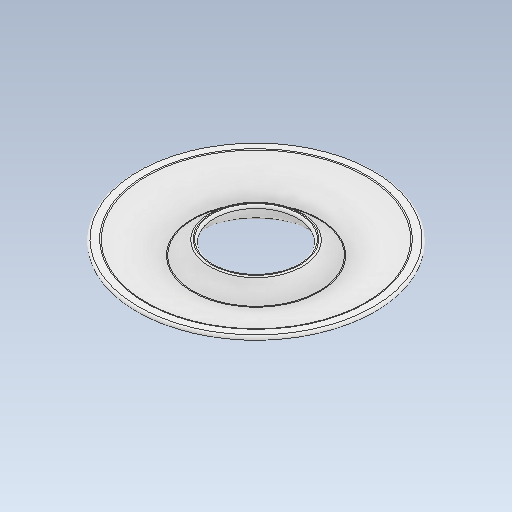
# Autodesk Inventor part: 8002_base_132uH_DCore_2layer_Tx_Filter_MPSv2_v1
Saved by Autodesk Inventor 2021 (Build 250183000, 183)
## iProperties
Created: 2021-02-24
Part Number: 8002_base_132uH_DCore_2layer_Tx_Filter_MPSv2_v1
Material: Acetal Resin, White
Document SubType Name: Modeling
Designer: Barksdale
Density: 1.425 g/cm^3
Appearance: Smooth - White
Author: Barksdale
Autodesk Inventor part; units mm, degrees
ref_plane "YZ Plane" through (0, 0, 0) normal (1, 0, 0) x (0, 1, 0)
ref_plane "XZ Plane" through (0, 0, 0) normal (0, 1, 0) x (-1, 0, 0)
ref_plane "XY Plane" through (0, 0, 0) normal (0, 0, 1) x (1, 0, 0)
sketch "Sketch1" plane through (0, 0, 0) normal (0, 0, 1) x (1, 0, 0)
  arc A0 (15.1396, -15.5997) -> (26.1298, -12.284) centre (15.0348, 4.6194) ccw
  arc A1 (11.0335, -12.4095) -> (14.937, -15.558) centre (18.7381, -6.8515) ccw
  arc A2 (9.9209, -12.8881) -> (14.937, -18.058) centre (18.7381, -9.3515) ccw
  arc A3 (15.1396, -18.0997) -> (28.3715, -13.0778) centre (15.0348, 2.1194) ccw
  line L0 (26.4042, -12.202) -> (28.0417, -12.202)
  line L1 (28.0417, -12.202) -> (26.2537, -12.202)
  line L2 (10.628, -12.202) -> (10.3849, -12.202)
  arc A4 (10.3849, -12.202) -> (9.9209, -12.8881) centre (10.3849, -12.702) ccw
  arc A5 (11.0335, -12.4095) -> (10.628, -12.202) centre (10.628, -12.702) ccw
  arc A6 (26.4042, -12.202) -> (26.1298, -12.284) centre (26.4042, -12.702) ccw
  arc A7 (28.3715, -13.0778) -> (28.0417, -12.202) centre (28.0417, -12.702) ccw
  arc A8 (14.937, -18.058) -> (15.1396, -18.0997) centre (15.137, -17.5997) ccw
  arc A9 (14.937, -15.558) -> (15.1396, -15.5997) centre (15.137, -15.0997) ccw
  line L3 (0, 0) -> (0, -18.0894)
  line L4 (15.137, -17.5997) -> (19.2939, -17.5997)
  line L5 (19.2939, -17.5997) -> (19.2939, -19.2305)
  line L6 (19.2939, -19.2305) -> (15.137, -19.2305)
  line L7 (15.137, -19.2305) -> (15.137, -17.5997)
  point P0 (9.6758, -12.202)
  point P1 (10.888, -12.202)
  point P2 (19.2939, -17.6463)
  point P3 (15.137, -18.0997)
  dimension "d1" = 0.5
  constraints: 23 point on circle, 16 end point, 12 tangent, 10 centre point, 5 equal radius, 3 point on line, 2 horizontal, 2 parallel, 1 perpendicular, 1 vertical
  measures "d1" radius of A4
revolve "Revolution2" add sketch "Sketch1" angle 360 about axis through (0, 0, 0) along (0, -1, 0)
fillet "Fillet5" radius 1 4 edges at (-15.137, -19.2305, 0) (-15.137, -18.0997, 0) (-19.2939, -19.2305, 0) (-19.2939, -17.6463, 0)
body "Solid2"
